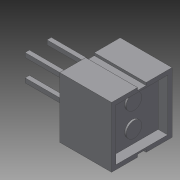
# Autodesk Inventor part: cny-70
Saved by Autodesk Inventor 2014 (Build 180170000, 170)
## iProperties
Created: 2013-09-05
Part Number: cny-70
Material: Generisch
Document SubType Name: Modeling
Designer: solidworks
Density: 1 g/cm^3
Appearance: Vorgabe
Author: solidworks
Autodesk Inventor part; units mm, degrees
ref_plane "YZ Plane" through (0, 0, 0) normal (1, 0, 0) x (0, 1, 0)
ref_plane "XZ Plane" through (0, 0, 0) normal (0, 1, 0) x (-1, 0, 0)
ref_plane "XY Plane" through (0, 0, 0) normal (0, 0, 1) x (1, 0, 0)
sketch "Skizze1" plane through (0, 0, 0) normal (1, 0, 0) x (0, 1, 0)
  line L0 (0, 0) -> (7, 0)
  line L1 (7, 0) -> (7, 7)
  line L2 (7, 7) -> (0, 7)
  line L3 (0, 7) -> (0, 0)
  line L4 (3, 7) -> (4, 7)
  line L5 (4, 7) -> (4, 6.7)
  line L6 (4, 6.7) -> (3, 6.7)
  line L7 (3, 6.7) -> (3, 7)
  line L8 (3, 0.3) -> (4, 0.3)
  line L9 (4, 0.3) -> (4, 0)
  line L10 (4, 0) -> (3, 0)
  line L11 (3, 0) -> (3, 0.3)
  dimension "d0" = 7
  dimension "d1" = 7
  dimension "d2" = 1
  dimension "d3" = 0.3
  dimension "d5" = 3
  constraints: 24 end point, 6 parallel, 3 collinear, 3 horizontal, 3 perpendicular, 2 equal length
  measures "d0" distance of L2.end L1.end
  measures "d1" distance of L1.end L0.end
  measures "d2" distance of L5.end L6.end
  measures "d3" distance between parallel lines of L2 L6
  measures "d5" distance between parallel lines of L3 L7
extrude "Extrusion1" add sketch "Skizze1" along normal blind 6 contours L3 L2 L7 L6 L5 L1 L0 L9 L8 L11
sketch "Skizze2" plane through (6, 0, 0) normal (1, 0, 0) x (0, 0, -1)
  line L0 (0, 7) -> (-7, 7) projected
  line L1 (-7, 7) -> (-7, 4) projected
  line L2 (-7, 0) -> (0, 0) projected
  line L3 (0, 0) -> (0, 3) projected
  line L4 (-6.5, 6.5) -> (-0.5, 6.5)
  line L5 (-0.5, 6.5) -> (-0.5, 0.5)
  line L6 (-0.5, 0.5) -> (-6.5, 0.5)
  line L7 (-6.5, 0.5) -> (-6.5, 6.5)
  dimension "d8" = 0.5
  dimension "d9" = 0.5
  dimension "d10" = 0.5
  dimension "d11" = 0.5
  constraints: 8 end point, 2 parallel, 1 horizontal, 1 perpendicular
  measures "d8" distance between parallel lines of L0 L4
  measures "d9" distance between parallel lines of L3 L5
  measures "d10" distance between parallel lines of L2 L6
  measures "d11" distance between parallel lines of L1 L7
extrude "Extrusion2" cut sketch "Skizze2" against normal blind 1.1
sketch "Skizze3" plane through (0, 0, 0) normal (-1, 0, 0) x (0, 0, 1)
  line L0 (7, 0) -> (0, 0) projected
  line L1 (0, 4) -> (0, 7) projected
  line L2 (1.98, 5.02) -> (2.48, 5.02)
  line L3 (2.48, 5.02) -> (2.48, 4.52)
  line L4 (2.48, 4.52) -> (1.98, 4.52)
  line L5 (1.98, 4.52) -> (1.98, 5.02)
  line L6 (4.52, 5.02) -> (5.02, 5.02)
  line L7 (5.02, 5.02) -> (5.02, 4.52)
  line L8 (5.02, 4.52) -> (4.52, 4.52)
  line L9 (4.52, 4.52) -> (4.52, 5.02)
  line L10 (1.98, 1.98) -> (2.48, 1.98)
  line L11 (2.48, 1.98) -> (2.48, 2.48)
  line L12 (2.48, 2.48) -> (1.98, 2.48)
  line L13 (1.98, 2.48) -> (1.98, 1.98)
  line L14 (4.52, 1.98) -> (5.02, 1.98)
  line L15 (5.02, 1.98) -> (5.02, 2.48)
  line L16 (5.02, 2.48) -> (4.52, 2.48)
  line L17 (4.52, 2.48) -> (4.52, 1.98)
  dimension "d14" = 0.5
  dimension "d15" = 0.5
  dimension "d16" = 0.5
  dimension "d17" = 0.5
  dimension "d18" = 0.5
  dimension "d19" = 0.5
  dimension "d20" = 0.5
  dimension "d21" = 0.5
  dimension "d24" = 1.98
  dimension "d25" = 3.04
  dimension "d26" = 3.04
  dimension "d27" = 1.98
  constraints: 32 end point, 8 parallel, 4 collinear, 4 horizontal, 4 perpendicular
  measures "d14" distance of L3.end L4.end
  measures "d15" distance of L2.end L3.end
  measures "d16" distance of L7.end L8.end
  measures "d17" distance of L6.end L7.end
  measures "d18" distance of L12.end L11.end
  measures "d19" distance of L11.end L10.end
  measures "d20" distance of L16.end L15.end
  measures "d21" distance of L15.end L14.end
  measures "d24" distance between parallel lines of L0 L10
  measures "d25" distance between parallel lines of L2 L10
  measures "d26" distance between parallel lines of L7 L5
  measures "d27" distance between parallel lines of L1 L5
extrude "Extrusion3" add sketch "Skizze3" along normal blind 6
sketch "Skizze4" plane through (4.9, 0, 0) normal (1, 0, 0) x (0, 0, -1)
  line L0 (-6.5, 0.5) -> (-6.5, 6.5) projected
  line L1 (-0.5, 0.5) -> (-6.5, 0.5) projected
  line L2 (-0.5, 6.5) -> (-0.5, 0.5) projected
  circle A0 centre (-4.9, 3.5) radius 0.9
  circle A1 centre (-2.1, 3.5) radius 0.9
  line L3 (-4.9, 3.5) -> (-2.1, 3.5)
  line L4 (-6.5, 6.5) -> (-0.5, 6.5) projected
  point P0 (0, 0)
  dimension "d30" = 1.8
  dimension "d31" = 1.8
  dimension "d32" = 2.8
  dimension "d33" = 3
  dimension "d34" = 1.6
  constraints: 2 centre point, 2 end point, 1 parallel, 1 perpendicular
  measures "d30" diameter of A0
  measures "d31" diameter of A1
  measures "d32" distance of L3.end L3.start
  measures "d33" distance between parallel lines of L1 L3
  measures "d34" distance from line of L0 L3.start
extrude "Extrusion4" add sketch "Skizze4" along normal blind 0.2 contours A0 | A1
